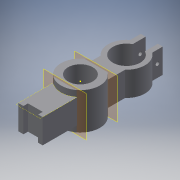
# Autodesk Inventor part: pen_holder_2
Saved by Autodesk Inventor 2016 (Build 200138000, 138)
## iProperties
Created: 2017-11-06
Part Number: pen_holder_2
Material: Generic
Document SubType Name: Modeling
Designer: Student
Density: 1 g/cm^3
Appearance: Default
Author: Student
Autodesk Inventor part; units mm, degrees
ref_plane "YZ Plane" through (0, 0, 0) normal (1, 0, 0) x (0, 1, 0)
ref_plane "XZ Plane" through (0, 0, 0) normal (0, 1, 0) x (-1, 0, 0)
sketch "Sketch1" plane through (0, 0, 0) normal (0, 1, 0) x (-1, 0, 0)
  circle A0 centre (0, 0) radius 5.25
  circle A1 centre (0, 0) radius 7.9375
  dimension "d0" = 10.5
  dimension "d1" = 2.6875
  constraints: 2 centre point, 1 coincident
  measures "d0" diameter of A0
  measures "d1" radial gap between concentric circles of A0 A1
extrude "Extrusion1" add sketch "Sketch1" along normal blind 15
ref_plane "Work Plane1" through (0, 0, 6.35) normal (0, 0, 1) x (1, 0, 0)
sketch "Sketch2" plane through (0, 0, 6.35) normal (0, 0, 1) x (1, 0, 0)
  line L0 (7.9375, 15) -> (-7.9375, 15) projected
  line L1 (-7.9375, 0) -> (7.9375, 0) projected
  line L2 (-5.0813, 12.5) -> (4.9187, 12.5)
  line L3 (4.9187, 12.5) -> (4.9187, 2.5)
  line L4 (4.9187, 2.5) -> (-5.0813, 2.5)
  line L5 (-5.0813, 2.5) -> (-5.0813, 12.5)
  point P0 (0, 0)
  dimension "d7" = 10
  dimension "d8" = 10
  constraints: 8 end point, 2 parallel, 1 horizontal, 1 perpendicular
  measures "d7" distance of L3.end L4.end
  measures "d8" distance of L2.end L3.end
extrude "Extrusion2" add sketch "Sketch2" along normal blind 15
ref_plane "Work Plane2" through (0, 0, -6.35) normal (0, 0, 1) x (1, 0, 0)
sketch "Sketch3" plane through (0, 0, -6.35) normal (0, 0, 1) x (1, 0, 0)
  line L0 (-5.25, 15) -> (5.25, 15) projected
  line L1 (5, 12.5) -> (-5, 12.5)
  line L2 (-5, 12.5) -> (-5, 2.5)
  line L3 (-5, 2.5) -> (5, 2.5)
  line L4 (5, 2.5) -> (5, 12.5)
  point P0 (0, 0)
  dimension "d14" = 10
  dimension "d15" = 10
  constraints: 8 end point, 2 parallel, 1 horizontal, 1 perpendicular
  measures "d14" distance of L3.end L2.end
  measures "d15" distance of L2.end L1.end
extrude "Extrusion3" add sketch "Sketch3" against normal blind 10
sketch "Sketch4" plane through (-5, 2.5, -6.35) normal (-1, 0, 0) x (0, 0, 1)
  point P0 (6.35, -2.5)
sketch "Sketch5" plane through (0, 12.5, 0) normal (0, 1, 0) x (1, 0, 0)
  line L0 (5, 6.35) -> (4.7625, 6.35) projected
  line L1 (5, 6.35) -> (5, 16.35)
  arc A0 (-4.5, 24.85) -> (4.5, 24.85) centre (0, 18.85) ccw
  arc A1 (-2.5, 23.8781) -> (2.5, 23.8781) centre (0, 18.85) ccw
  line L2 (-2.5, 29.1708) -> (-2.5, 23.8781)
  line L3 (2.5, 16.3221) -> (2.5, 16.35)
  line L4 (2.5, 23.8781) -> (2.5, 29.1708)
  line L5 (-4.5, 29.1708) -> (-4.5, 24.9936)
  line L6 (4.5, 24.9936) -> (4.5, 29.1708)
  line L7 (4.5, 24.9936) -> (4.5, 24.85)
  line L8 (-4.5, 24.9936) -> (-4.5, 24.85)
  line L9 (2.5, 29.1708) -> (4.5, 29.1708)
  line L10 (-2.5, 29.1708) -> (-4.5, 29.1708)
  point P0 (0, 0)
  dimension "d19" = 5
  dimension "d20" = 2
  constraints: 20 end point, 4 point on circle, 3 vertical, 2 centre point, 1 parallel, 1 perpendicular, 1 point on line
  measures "d19" distance of L4.end L2.start
  measures "d20" distance between parallel lines of L4 L6
extrude "Extrusion4" add sketch "Sketch5" against normal blind 10
sketch "Sketch6" plane through (0, 12.5, 0) normal (0, 1, 0) x (1, 0, 0)
  arc A0 (-2.5, 23.8781) -> (-5, 16.2942) centre (0, 18.85) ccw construction
  arc A1 (-2.5, 23.8781) -> (-5, 16.2942) centre (0, 18.85) ccw projected
  circle A2 centre (0, 18.85) radius 5.6153
  point P0 (0, 0)
  constraints: 1 coincident, 3 other
extrude "Extrusion5" cut sketch "Sketch6" against normal blind 10
sketch "Sketch7" plane through (4.5, 12.5, -24.85) normal (1, 0, 0) x (0, 0, -1)
  line L0 (0, 0) -> (4.3208, 0) construction
  line L1 (0, 0) -> (0, -10) construction
  line L2 (4.3208, -10) -> (0, -10) construction
  line L3 (4.3208, 0) -> (4.3208, -10) construction
  circle A0 centre (2.1604, -5) radius 0.75
  point P0 (-24.85, -12.5)
  dimension "d25" = 1.5
  constraints: 1 centre point
  measures "d25" diameter of A0
extrude "Extrusion6" cut sketch "Sketch7" against normal up to surface (9 mm away)
sketch "Sketch8" plane through (0, 12.5, 0) normal (0, 1, 0) x (1, 0, 0)
  arc A0 (-4.7625, -6.35) -> (4.7625, -6.35) centre (0, 0) ccw construction
  line L0 (-5.0813, -6.35) -> (-4.7625, -6.35) construction
  line L1 (-5.0813, -6.35) -> (-5.0813, -21.35) construction
  line L2 (4.9187, -21.35) -> (-5.0813, -21.35) construction
  line L3 (4.9187, -6.35) -> (4.9187, -21.35) construction
  line L4 (4.7625, -6.35) -> (4.9187, -6.35) construction
sketch "Sketch9" plane through (0, 15, 0) normal (0, 1, 0) x (1, 0, 0)
  circle A0 centre (0, 0) radius 5.25 projected
  circle A1 centre (0, 0) radius 5.05
  circle A2 centre (0, 0) radius 5.25
  dimension "d28" = 10.1
  constraints: 2 centre point, 2 coincident
  measures "d28" diameter of A1
extrude "Extrusion7" add sketch "Sketch9" against normal blind 15
sketch "Sketch10" plane through (0, 12.5, 0) normal (0, 1, 0) x (1, 0, 0)
  line L0 (4.9187, -6.35) -> (4.9187, -21.35) projected
  line L1 (4.9187, -21.35) -> (4.9187, -20.35)
  line L2 (4.9187, -20.35) -> (-5.0813, -20.35)
  line L3 (-5.0813, -6.35) -> (-5.0813, -21.35) projected
  line L4 (-5.0813, -21.35) -> (-5.0813, -20.35)
  line L5 (-5.0813, -21.35) -> (4.9187, -21.35)
  point P0 (0, 0)
  dimension "d31" = 1
  constraints: 8 end point, 2 perpendicular, 2 point on line, 1 collinear
  measures "d31" distance of L0.end L1.end
extrude "Extrusion8" cut sketch "Sketch10" against normal blind 15
sketch "Sketch11" plane through (0, 2.5, 0) normal (0, -1, 0) x (1, 0, 0)
  line L0 (-2.428, 18.5096) -> (2.572, 18.4901)
  line L1 (2.572, 18.4901) -> (2.822, 18.4901)
  line L2 (-2.428, 18.5096) -> (-2.678, 18.5096)
  line L3 (-2.678, 20.35) -> (2.822, 20.35)
  line L4 (-2.678, 18.5096) -> (-2.678, 20.35)
  line L5 (2.822, 18.4901) -> (2.822, 20.35)
  point P0 (0, 0)
  dimension "d35" = 0.25
  dimension "d38" = 0.25
  constraints: 12 end point, 2 horizontal, 1 other
  measures "d35" distance of L0.start L2.end
  measures "d38" distance of L0.end L1.end
extrude "Extrusion9" cut sketch "Sketch11" against normal up to next
equation "\"d35\" = d38"
body "Solid1"
